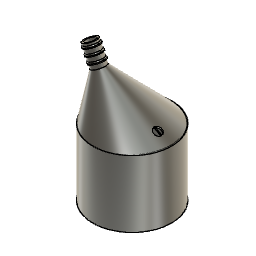
goutière (Autodesk Fusion 360 design; units mm, degrees)
Autodesk Fusion 360 part; units mm, degrees
sketch "Esquisse1" plane through (0, 0, 0) normal (0, 0, 1) x (1, 0, 0)
  circle A0 centre (0, 0) radius 6.75
  line L0 (-43.5, 0.0359) -> (-6.7499, 0.0359)
  line L1 (6.7499, 0.0359) -> (43.5, 0.0359)
  circle A1 centre (0, 0) radius 5.5
  circle A2 centre (0, 0.0001) radius 7.375
  line L2 (-42.7583, -14.0259) -> (-41.1767, -14.0259)
  line L3 (-42.3762, 15.1412) -> (-40.7799, 15.1412)
  dimension "d1" = 13.5
  dimension "d18" = 11
  dimension "d19" = 14.75
  constraint coincident A0 L0.end
  constraint horizontal L0
  constraint coincident A0 L1.start
  constraint parallel L0 L1
  constraint concentric A0 A1
  constraint horizontal L2
  constraint parallel L2 L3
  measures "d1" diameter of A0
  measures "d18" diameter of A1
  measures "d19" diameter of A2
extrude "Extrusion1" add sketch "Esquisse1" along normal blind 20 from surface at 3 contours A0 | A1 makes body 1
move_body "Déplacer1" bodies 1 to x (1, 0, 0) y (0, 1, 0) z (0, 0, 1) at (0, 0, 35)
extrude "Extrusion6" add sketch "Esquisse1" along normal blind 2 from surface at 48 contours A0 L0 L1 A2 | A0 L0 L1 A2 bodies 1
extrude "Extrusion7" add sketch "Esquisse1" along normal blind 2 from surface at 54 contours A0 L0 L1 A2 | A0 L0 L1 A2 bodies 1
extrude "Extrusion8" add sketch "Esquisse1" along normal blind 2 from surface at 42 contours A0 L0 L1 A2 | A0 L0 L1 A2 bodies 1
fillet "Congé1" radius 1.5 3 edges at (-6.8759, -2.6668, 50) (-6.8759, -2.6668, 56) (-6.8759, -2.6668, 44) on bodies 1
move_body "Déplacer2" bodies 1 to x (1, 0, 0) y (0, 1, 0) z (0, 0, 1) at (0, 0, -40)
sketch "Esquisse9" plane through (0, 0, -2) normal (0, 0, -1) x (1, 0, 0)
  circle A0 centre (0, 0) radius 37.5
  circle A1 centre (0, 0) radius 38.375
  circle A2 centre (0, 0) radius 6.75
  line L0 (-6.75, 0) -> (6.75, 0)
  line L1 (0, -6.75) -> (0, 6.75)
  dimension "d66" = 75
  dimension "d67" = 76.75
  constraint coincident A0.centre A1.centre
  constraint concentric A0 A1
  constraint coincident A2 L1.end
  constraint coincident A2 L1.start
  constraint coincident A2 L0.start
  constraint coincident A2 L0.end
  measures "d66" diameter of A0
  measures "d67" diameter of A1
extrude "Extrusion17" add sketch "Esquisse9" 1 faces at (-1.125, 1.9486, -2) along normal blind 2 from surface at 35 separate body contours A0 | A1 on bodies 1 makes body 2
extrude "Extrusion15" add sketch "Esquisse9" along normal blind 65 from surface at 35 separate body contours A1 makes body 3
move_body "Déplacer3" bodies 1 to x (1, 0, 0) y (0, 1, 0) z (0, 0, 1) at (-30.9948, 0.2409, -22.1468)
sketch "Esquisse10" plane through (0, 0, 0) normal (0, 0, 1) x (1, 0, 0)
  line L0 (0, 5) -> (5, 5)
  line L1 (5, 5) -> (5, -5)
  line L2 (5, -5) -> (0, -5)
  line L3 (0, -5) -> (0, 5)
  constraint horizontal L0
  constraint vertical L1
  constraint horizontal L2
  constraint vertical L3
extrude "Extrusion16" add sketch "Esquisse10" along normal blind 10 separate body makes body 4
move_body "Déplacer4" bodies 1 to x (0.906308, 0, 0.422618) y (0, 1, 0) z (-0.422618, 0, 0.906308) at (4.2262, 0, 0.9369)
move_body "Déplacer5" bodies 1 to x (1, 0, 0) y (0, 1, 0) z (0, 0, 1) at (-19, 0, 29)
sketch "Esquisse11" plane through (-3.9003, 0, 8.3642) normal (0.422618, 0, -0.906308) x (0, 1, 0)
  circle A0 centre (0.2409, -31.7326) radius 6.75
  circle A1 centre (0.2409, -31.7326) radius 6.75
  constraint concentric A0 A1
loft "Lissage3" add section 1 face at (-32.5603, 1.7048, -5.0002) section 2 face at (0.9559, -12.7559, -37) separate body on bodies 1 2 makes body 5
shell "Coque5" thickness 1.75 removed faces 1 at (0.9559, -12.7559, -37) on bodies 5
hole "Perçage3" at (25.8707, -0.857, -30.3044) direction (-0.472361, 0.01359, -0.8813) diameter 8 depth 8 tip angle 180 bodies 5
hole "Perçage4" at (-41.1121, 0.2409, 13.0796) direction (0.422618, 0, -0.906308) diameter 9.8 depth 9.8 tip angle 180 bodies 1
extrude "Extrusion18" cut 1 faces at (-39.3553, 1.2736, 3.0858) along direction (0.422618, 0, -0.906308) blind 35 on bodies 1 bodies 1 5
hidden bodies 4 2
